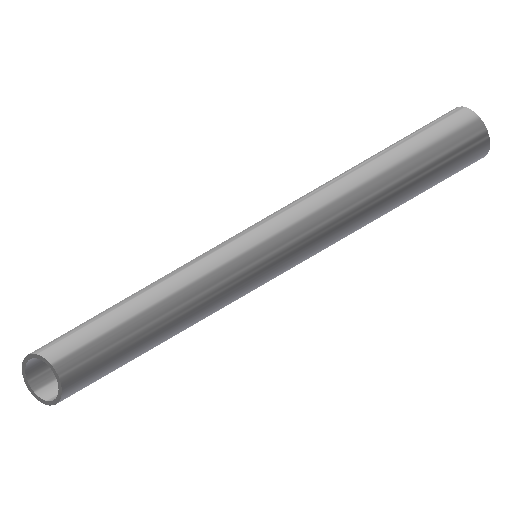
# Autodesk Inventor part: cutoff pipe
Saved by Autodesk Inventor 2022 (Build 260148000, 148)
## iProperties
Created: 2007-05-11
Part Number: cutoff pipe
Material: Steel, Mild
Document SubType Name: Modeling
Designer: LionelF
Density: 7.86 g/cm^3
Mass: 1517.66 g
Surface Area: 1094.6 cm^2
Volume: 193.086 cm^3
Appearance: Steel
Author: LionelF
Autodesk Inventor part; units mm, degrees
ref_plane "YZ Plane" through (0, 0, 0) normal (1, 0, 0) x (0, 1, 0)
ref_plane "XZ Plane" through (0, 0, 0) normal (0, 1, 0) x (-1, 0, 0)
ref_plane "XY Plane" through (0, 0, 0) normal (0, 0, 1) x (1, 0, 0)
sketch "Sketch1" plane through (0, 0, 0) normal (0, 0, 1) x (1, 0, 0)
  circle A0 centre (0, 0) radius 21.082
  circle A1 centre (0, 0) radius 17.526
  dimension "d0" = 42.164
  dimension "d1" = 35.052
  constraints: 2 centre point, 1 coincident
  measures "d0" diameter of A0
  measures "d1" diameter of A1
extrude "Extrusion1" add sketch "Sketch1" along normal blind 447.675
body "Solid1"
